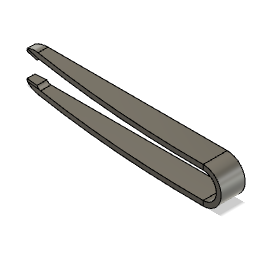
Tweezers v08222021_1309 (Autodesk Fusion 360 design; units mm, degrees)
Autodesk Fusion 360 part; units mm, degrees
sketch "Sketch1" plane through (0, 0, 0) normal (0, 0, 1) x (1, 0, 0)
  line L0 (-40, 7.5) -> (40, 7.5)
  line L1 (40, -7.5) -> (-40, -7.5)
  line L2 (-40, 7.5) -> (40, -7.5) construction
  line L3 (40, 7.5) -> (-40, -7.5) construction
  arc A0 (40, -7.5) -> (40, 7.5) centre (40, 0) ccw
  arc A1 (40, -5.5) -> (40, 5.5) centre (40, 0) ccw
  line L4 (-35, 5.5) -> (40, 5.5)
  line L5 (40, -5.5) -> (-29.3333, -5.5)
  line L6 (-40, -7.5) -> (-40, -5.9374)
  line L7 (-40, 5.9374) -> (-40, 7.5)
  line L8 (-35, 5.5) -> (-40, 5.9374)
  line L9 (-29.3333, -5.5) -> (-35, -5.5)
  line L10 (-35, -5.5) -> (-40, -5.9374)
  dimension "d1" = 80
  dimension "d2" = 15
  constraint horizontal L0
  constraint parallel L0 L1
  constraint coincident L2 origin
  constraint coincident L3 origin
  constraint tangent L1 A0
  constraint concentric A0 A1
  constraint parallel L0 L4
  constraint parallel L1 L5
  constraint tangent A1 L4
  constraint tangent A1 L5
  constraint collinear L6 L7
  constraint coincident L3 L5.end
  constraint parallel L1 L9
  measures "d1" distance of L1.start L1.end
  measures "d2" distance of L0.end L1.start
sketch "Sketch2" plane through (0, 0, 0) normal (0, 1, 0) x (1, 0, 0)
sketch "Sketch3" plane through (0, 0, 0) normal (0, 0, 1) x (1, 0, 0)
extrude "Extrude1" add sketch "Sketch1" along normal blind 10
sketch "Sketch4" plane through (0, -7.5, 0) normal (0, -1, 0) x (1, 0, 0)
  line L0 (-40, 0) -> (40, 0)
  line L1 (40, 0) -> (40, 10)
  line L2 (40, 10) -> (-40, 10)
  line L3 (-40, 10) -> (-40, 0)
  line L4 (-40, 0) -> (-40, 10)
  line L5 (-40, 10) -> (40, 10)
  line L6 (40, 0) -> (-40, 0)
  arc A0 (40, 10) -> (-40, 3.2305) centre (40, -466.0962) ccw
  point P0 (-40, 3.2305)
  point P1 (-40, 3)
  dimension "d9" = 3
  constraint coincident L4 P0
  constraint tangent L5 A0
  constraint coincident L1.end L2.start
  constraint coincident P0 A0.end
  measures "d9" distance of L0.start P1
extrude "Extrude2" cut sketch "Sketch4" against normal blind 19 contours L2 L3 L4 L5 A0
extrude "Extrude3" add 1 faces at (-37.5004, 5.7188, 1.2166) along direction (-0.087156, -0.996195, 0) blind 1
extrude "Extrude4" add 1 faces at (-37.5004, -5.7188, 1.2166) along direction (-0.087156, 0.996195, 0) blind 1
fillet "Fillet1" radius 2 2 edges at (-35, 5.5, 2.0277) (-35, -5.5, 2.0277)
fillet "Fillet2" radius 10 2 edges at (-40, 7.5, 1.6153) (-40, -7.5, 1.6153)
